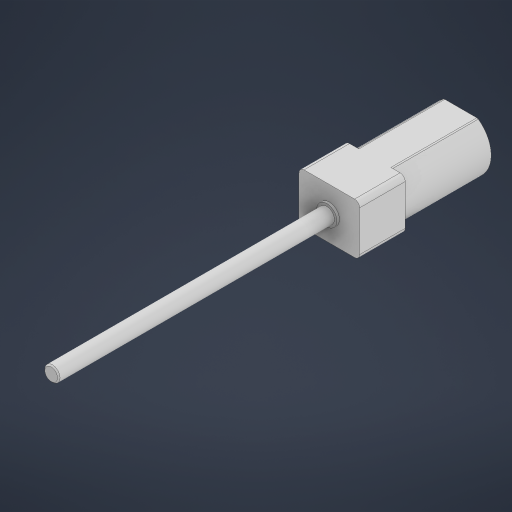
# Autodesk Inventor part: DC Motor
Saved by Autodesk Inventor 2023.4 (Build 274418000, 418)
## iProperties
Created: 2023-11-07
Part Number: DC Motor
Material: Generic
Document SubType Name: Modeling
Designer: xSibe
Density: 1 g/cm^3
Appearance: Default
Author: xSibe
Autodesk Inventor part; units mm, degrees
ref_plane "YZ Plane" through (0, 0, 0) normal (1, 0, 0) x (0, 1, 0)
ref_plane "XZ Plane" through (0, 0, 0) normal (0, 1, 0) x (-1, 0, 0)
ref_plane "XY Plane" through (0, 0, 0) normal (0, 0, 1) x (1, 0, 0)
sketch "Sketch1" plane through (0, 0, 0) normal (0, 0, 1) x (1, 0, 0)
  line L0 (-6, -5) -> (6, -5)
  line L1 (6, -5) -> (6, 5)
  line L2 (6, 5) -> (-6, 5)
  line L3 (-6, 5) -> (-6, -5)
  line L4 (-6, -5) -> (6, 5) construction
  line L5 (6, -5) -> (-6, 5) construction
  point P0 (0, 0)
  dimension "d0" = 12
  dimension "d1" = 10
  constraints: 12 end point, 2 midpoint, 2 parallel, 1 horizontal, 1 perpendicular
  measures "d0" distance of L2.end L1.end
  measures "d1" distance of L1.end L0.end
extrude "Extrusion1" add sketch "Sketch1" along normal mid plane 26
sketch "Sketch2" plane through (0, 0, 13) normal (0, 0, 1) x (1, 0, 0)
  circle A0 centre (0, 0) radius 1.5
  circle A1 centre (0, 0) radius 2
  dimension "d4" = 3
  dimension "d12" = 4
  constraints: 2 centre point, 2 coincident
  measures "d4" diameter of A0
  measures "d12" diameter of A1
extrude "Extrusion2" add sketch "Sketch2" along normal blind 55 contours A0
fillet "Fillet1" radius 1 4 edges at (6, 5, 0) (-6, 5, 0) (6, -5, 0) (-6, -5, 0)
sketch "Sketch3" plane through (0, 0, -13) normal (0, 0, -1) x (-1, 0, 0)
  arc A0 (5, -5) -> (6, -4) centre (5, -4) ccw projected
  line L0 (6, -4) -> (6, 4) projected
  arc A1 (6, 4) -> (5, 5) centre (5, 4) ccw projected
  line L1 (5, 5) -> (-5, 5) projected
  arc A2 (-5, 5) -> (-6, 4) centre (-5, 4) ccw projected
  line L2 (-6, 4) -> (-6, -4) projected
  arc A3 (-6, -4) -> (-5, -5) centre (-5, -4) ccw projected
  line L3 (-5, -5) -> (5, -5) projected
  circle A4 centre (0, 0) radius 6
  point P0 (3.3166, 5)
  point P1 (6, 0)
  point P2 (3.3166, -5)
  point P3 (-3.3166, -5)
  point P4 (-6, 0)
  point P5 (-3.3166, 5)
  dimension "d8" = 12
  constraints: 1 centre point, 1 coincident
  measures "d8" diameter of A4
extrude "Extrusion3" cut sketch "Sketch3" against normal blind 17 contours L3 A4 L0 A0 | A4 L1 A1 L0 | L3 A3 L2 A4 | L2 A2 L1 A4
fillet "Fillet2" radius 0.5 4 edges at (-3.3166, -5, -4.5) (3.3166, -5, -4.5) (-3.3166, 5, -4.5) (3.3166, 5, -4.5)
extrude "Extrusion4" add sketch "Sketch2" along normal blind 0.5
chamfer "Chamfer1" distance 0.25 angle 45 1 edges at (-1.5, 0, 68)
body "Solid1"
